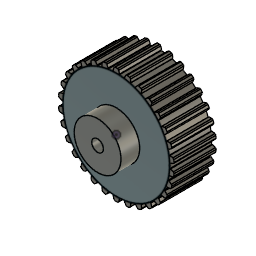
Assembly (Autodesk Fusion 360 archive; units mm, degrees)
design "Gear(30)"
part number: 2026-07-17-20-20-12-851
Autodesk Fusion 360 part; units mm, degrees
sketch "Sketch1" plane through (0, 0, 0) normal (0, 1, 0) x (1, 0, 0)
  circle A0 centre (0, 0) radius 22.8
  dimension "d1" = 45.6
  constraint coincident A0.centre origin
  measures "d1" diameter of A0
extrude "Extrude1" add sketch "Sketch1" along normal blind 18 makes body 1
sketch "Sketch2" plane through (0, 0, 0) normal (0, -1, 0) x (1, 0, 0)
  circle A0 centre (0, 0) radius 22.8
  circle A1 centre (0, 0) radius 2.5
  dimension "d4" = 5
  constraint concentric A0 A1
  measures "d4" diameter of A1
extrude "Extrude2" cut sketch "Sketch2" against normal blind 65 contours A1 bodies 1
sketch "Sketch3" plane through (0, 0, 0) normal (0, -1, 0) x (1, 0, 0)
  circle A0 centre (0, 0) radius 2.5
  circle A1 centre (0, 0) radius 22.8
  circle A2 centre (0, 0) radius 10
  dimension "d7" = 20
  constraint coincident A0.centre A1.centre
  measures "d7" diameter of A2
extrude "Extrude3" add sketch "Sketch3" along normal blind 8 contours A2 bodies 1
sketch "Sketch5" plane through (0, 18, 0) normal (0, 1, 0) x (-1, 0, 0)
  circle A0 centre (0, 0) radius 2.5
  circle A1 centre (0, 0) radius 22.8
  circle A2 centre (0, 0) radius 22.8
  line L0 (-1.3883, 23.1344) -> (-1.0229, 24.3903)
  line L1 (-1.1003, 22.7506) -> (1.0933, 22.7506)
  line L2 (-0.5435, 24.7506) -> (0.5131, 24.7506)
  line L3 (0.9908, 24.3982) -> (1.3799, 23.1392)
  arc A3 (-0.5435, 24.7506) -> (-1.0229, 24.3903) centre (-0.5428, 24.2506) ccw
  arc A4 (0.9908, 24.3982) -> (0.5131, 24.7506) centre (0.5131, 24.2506) ccw
  arc A5 (-1.3883, 23.1344) -> (-1.1003, 22.7506) centre (-1.1003, 23.0506) ccw
  arc A6 (1.0933, 22.7506) -> (1.3799, 23.1392) centre (1.0933, 23.0506) ccw
  point P0 (-1.5, 22.7506)
  point P1 (-0.918, 24.7506)
  point P2 (1.5, 22.7506)
  point P3 (0.882, 24.7506)
  dimension "d28" = 3
  dimension "d29" = 1.8
  dimension "d31" = 2
  dimension "d32" = 0.5
  dimension "d33" = 0.5
  dimension "d34" = 0.3
  constraint coincident A2 P0
  constraint horizontal L1
  constraint horizontal L2
  constraint coincident A2 P2
  constraint coincident P1 L0
  constraint coincident P1 L2
  constraint tangent L0 A3
  constraint coincident P3 L2
  constraint coincident P3 L3
  constraint tangent L2 A4
  constraint tangent L3 A4
  constraint coincident P0 L0
  constraint coincident P0 L1
  constraint tangent L0 A5
  constraint tangent L1 A5
  constraint coincident P2 L1
  constraint coincident P2 L3
  constraint tangent L1 A6
  constraint tangent L3 A6
  constraint equal A5 A6
  measures "d28" distance of P0 P2
  measures "d29" distance of P1 P3
  measures "d31" distance of L1 L2
  measures "d32" radius of A3
  measures "d33" radius of A4
  measures "d34" radius of A5
extrude "Extrude7" add sketch "Sketch5" against normal blind 18 separate body contours A1 A2 L0 L2 L3 A3 A4 A5 A6 makes body 2
pattern_circular "C-Pattern3" count 30 over 360 about axis through (0, 18, 0) along (0, -1, 0) of "Extrude7" makes body 3 at (-3.8213, 6, 22.4775) makes body 4 at (-9.3924, 6, 20.7755) makes body 5 at (-13.5066, 6, 18.3688) makes body 6 at (-16.3034, 6, 15.9386) makes body 7 at (-19.8102, 6, 11.287) makes body 8 at (-21.6416, 6, 7.1751) makes body 9 at (-22.6883, 6, 2.2537) makes body 10 at (-22.6611, 6, -2.5127) makes body 11 at (-21.6435, 6, -7.1693) makes body 12 at (-20.1965, 6, -10.5802) makes body 13 at (-16.8563, 6, -15.3527) makes body 14 at (-14.1471, 6, -17.8801) makes body 15 at (-9.1545, 6, -20.8815) makes body 16 at (-5.6515, 6, -22.0885) makes body 17 at (0.1302, 6, -22.7996) makes body 18 at (4.8677, 6, -22.2743) makes body 19 at (9.3924, 6, -20.7755) makes body 20 at (12.6333, 6, -18.98) makes body 21 at (16.3034, 6, -15.9386) makes body 22 at (19.8102, 6, -11.287) makes body 23 at (21.6416, 6, -7.1751) makes body 24 at (22.6883, 6, -2.2537) makes body 25 at (22.6611, 6, 2.5127) makes body 26 at (21.6435, 6, 7.1693) makes body 27 at (20.1965, 6, 10.5802) makes body 28 at (16.8563, 6, 15.3527) makes body 29 at (14.1471, 6, 17.8801) makes body 30 at (10.1205, 6, 20.4308) makes body 31 at (5.6515, 6, 22.0885)

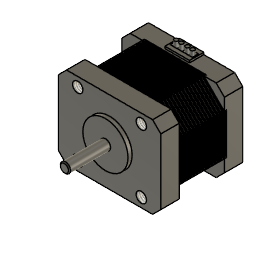
design "conveyor_belt_Assembly"
part number: 2026-07-17-14-44-36-904
Autodesk Fusion 360 part; units mm, degrees
sketch "Sketch1" plane through (0, 0, 0) normal (0, 0, 1) x (1, 0, 0)
  line L0 (25, -20) -> (-25, -20)
  line L1 (-25, -20) -> (-25, 20)
  line L2 (-25, 20) -> (25, 20)
  line L3 (25, 20) -> (25, -20)
  line L4 (25, -20) -> (-25, 20) construction
  line L5 (-25, -20) -> (25, 20) construction
  dimension "d1" = 50
  dimension "d2" = 40
  constraint horizontal L0
  constraint perpendicular L0 L1
  constraint parallel L0 L2
  constraint parallel L1 L3
  constraint coincident L4 origin
  constraint coincident L5 origin
  measures "d1" distance of L1.end L2.end
  measures "d2" distance of L0.end L1.end
extrude "Extrude1" add sketch "Sketch1" along normal blind 40
chamfer "Chamfer1" distance 4 angle 45 4 edges at (25, 0, 40) (25, 0, 0) (-25, 0, 40) (-25, 0, 0)
sketch "Sketch2" plane through (0, -20, 0) normal (0, -1, 0) x (1, 0, 0)
  line L0 (-25, 4) -> (-21, 0)
  line L1 (-21, 0) -> (21, 0)
  line L2 (21, 0) -> (25, 4)
  line L3 (25, 4) -> (25, 36)
  line L4 (25, 36) -> (21, 40)
  line L5 (21, 40) -> (-21, 40)
  line L6 (-21, 40) -> (-25, 36)
  line L7 (-25, 36) -> (-25, 4)
  circle A0 centre (0, 20) radius 2.5
  dimension "d6" = 40
  dimension "d7" = 5
  dimension "d8" = 20
  measures "d6" distance of L1 L5
  measures "d7" diameter of A0
  measures "d8" distance of origin A0.centre
extrude "Extrude2" add sketch "Sketch2" along normal blind 22 contours A0
sketch "Sketch3" plane through (0, -20, 0) normal (0, -1, 0) x (1, 0, 0)
  circle A0 centre (0, 20) radius 2.5
  line L0 (-25, 4) -> (-21, 0)
  line L1 (-21, 0) -> (21, 0)
  line L2 (21, 0) -> (25, 4)
  line L3 (25, 4) -> (25, 36)
  line L4 (25, 36) -> (21, 40)
  line L5 (21, 40) -> (-21, 40)
  line L6 (-21, 40) -> (-25, 36)
  line L7 (-25, 36) -> (-25, 4)
  circle A1 centre (0, 20) radius 11
  dimension "d12" = 22
  constraint concentric A0 A1
  measures "d12" diameter of A1
extrude "Extrude3" add sketch "Sketch3" along normal blind 2 contours A1
sketch "Sketch4" plane through (0, -20, 0) normal (0, -1, 0) x (1, 0, 0)
  circle A0 centre (0, 20) radius 11
  line L0 (-25, 4) -> (-21, 0)
  line L1 (-21, 0) -> (21, 0)
  line L2 (21, 0) -> (25, 4)
  line L3 (25, 4) -> (25, 36)
  line L4 (25, 36) -> (21, 40)
  line L5 (21, 40) -> (-21, 40)
  line L6 (-21, 40) -> (-25, 36)
  line L7 (-25, 36) -> (-25, 4)
  circle A1 centre (-15.5, 35.5) radius 2
  circle A2 centre (-15.5, 4.5) radius 2
  circle A3 centre (15.5, 4.5) radius 2
  circle A4 centre (15.5, 35.5) radius 2
  dimension "d15" = 4
  dimension "d16" = 15.5
  dimension "d17" = 15.5
  dimension "d19" = 360
  measures "d15" diameter of A1
  measures "d16" vertical distance of A0.centre A1.centre
  measures "d17" horizontal distance of A0.centre A1.centre
sketch "Sketch5" plane through (0, 20, 0) normal (0, 1, 0) x (-1, 0, 0)
  line L0 (21, 0) -> (25, 4)
  line L1 (25, 4) -> (25, 36)
  line L2 (25, 36) -> (21, 40)
  line L3 (21, 40) -> (-21, 40)
  line L4 (-21, 40) -> (-25, 36)
  line L5 (-25, 36) -> (-25, 4)
  line L6 (-25, 4) -> (-21, 0)
  line L7 (-21, 0) -> (21, 0)
  line L8 (-25, 30) -> (-15, 40)
  line L9 (-25, 30) -> (-25, 40)
  line L10 (-25, 40) -> (-15, 40)
  line L11 (25, 10) -> (15, 0)
  line L12 (25, 0) -> (15, 0)
  line L13 (25, 10) -> (25, 0)
  line L14 (-25, 10) -> (-15, 0)
  line L15 (-25, 10) -> (-25, 0)
  line L16 (-25, 0) -> (-15, 0)
  line L17 (25, 40) -> (15, 40)
  line L18 (25, 30) -> (25, 40)
  line L19 (25, 30) -> (15, 40)
  point P0 (0, 20)
  dimension "d20" = 10
  dimension "d21" = 10
  dimension "d22" = 20
  dimension "d25" = 10
  dimension "d26" = 10
  constraint coincident L5 L8.start
  constraint coincident L3 L8.end
  constraint parallel L5 L9
  constraint coincident L5 L14.start
  constraint coincident L7 L14.end
  constraint parallel L5 L15
  constraint perpendicular L15 L16
  measures "d20" distance of L3 L8.start
  measures "d21" distance of L5 L8.end
  measures "d22" distance of origin P0
  measures "d25" distance of L7 L14.start
  measures "d26" distance of L5 L14.end
extrude "Extrude4" cut sketch "Sketch5" against normal blind 22 from surface at -9 contours L0 L1 L7 L11 L12 L13 | L0 L12 L13 | L5 L6 L7 L14 L15 L16 | L1 L2 L3 L17 L18 L19 | L6 L15 L16 | L2 L17 L18 | L3 L4 L5 L8 L9 L10 | L4 L9 L10
sketch "Sketch6" plane through (0, 11, 0) normal (0, -1, 0) x (1, 0, 0)
  line L0 (25, 36) -> (21, 40)
  line L1 (21, 40) -> (15, 40)
  line L2 (15, 40) -> (25, 30)
  line L3 (25, 30) -> (25, 36)
  line L4 (-25, 10) -> (-15, 0)
  line L5 (-15, 40) -> (15, 40)
  line L6 (-25, 10) -> (-25, 30)
  line L7 (25, 10) -> (15, 0)
  line L8 (25, 30) -> (15, 40)
  line L9 (-15, 0) -> (15, 0)
  line L10 (15, 0) -> (25, 10)
  line L11 (25, 30) -> (25, 10)
  line L12 (25, 30) -> (15, 40)
  line L13 (-15, 40) -> (-25, 30)
  line L14 (-14.7929, 39.5) -> (14.7929, 39.5)
  line L15 (24.5, 29.7929) -> (14.7929, 39.5)
  line L16 (24.5, 29.7929) -> (24.5, 10.2071)
  line L17 (14.7929, 0.5) -> (24.5, 10.2071)
  line L18 (-14.7929, 0.5) -> (14.7929, 0.5)
  line L19 (-24.5, 10.2071) -> (-14.7929, 0.5)
  line L20 (-24.5, 10.2071) -> (-24.5, 29.7929)
  line L21 (-14.7929, 39.5) -> (-24.5, 29.7929)
  dimension "d42" = -0.5
  constraint coincident L4.start L6.start
  constraint coincident L4.end L9.start
  constraint coincident L7.end L9.end
  constraint coincident L7.start L10.end
  constraint coincident L2.end L3.start
  constraint coincident L1.end L2.start
  constraint perpendicular L2 L13
extrude "Extrude7" cut sketch "Sketch6" against normal blind 1 contours L2 L4 L5 L6 L7 L8 L9 L10 L11 L12 L13
pattern_linear "R-Pattern2" count 16 spacing 1.4667 along (0, -1, 0) of "Extrude7"
sketch "Sketch7" plane through (0, 0, 40) normal (0, 0, 1) x (-1, 0, 0)
  line L0 (15, -11) -> (15, -12)
  line L1 (15, -12) -> (-15, -12)
  line L2 (-15, -12) -> (-15, -11)
  line L3 (-15, -11) -> (-21, -11)
  line L4 (-21, -11) -> (-21, -20)
  line L5 (-21, -20) -> (21, -20)
  line L6 (21, -20) -> (21, -11)
  line L7 (21, -11) -> (15, -11)
  line L8 (0, -20) -> (0, -13) construction
  line L9 (-6, -20) -> (6, -20)
  line L10 (6, -20) -> (6, -13)
  line L11 (6, -13) -> (-6, -13)
  line L12 (-6, -13) -> (-6, -20)
  line L13 (-6, -20) -> (6, -13) construction
  line L14 (6, -20) -> (-6, -13) construction
  point P0 (0, -16.5)
  dimension "d49" = 12
  constraint midpoint L5 L8.start
  constraint perpendicular L5 L8
  constraint horizontal L9
  constraint perpendicular L9 L10
  constraint parallel L9 L11
  constraint parallel L10 L12
  constraint coincident L13 P0
  constraint coincident L14 P0
  constraint midpoint L8 P0
  measures "d49" distance of L10.end L11.end
extrude "Extrude8" add sketch "Sketch7" along normal blind 1 contours L5 L9 L10 L11 L12
sketch "Sketch8" plane through (0, 0, 41) normal (0, 0, 1) x (-1, 0, 0)
  line L0 (-6, -13) -> (-6, -20)
  line L1 (-6, -20) -> (6, -20)
  line L2 (6, -20) -> (6, -13)
  line L3 (6, -13) -> (-6, -13)
  line L4 (0, -20) -> (0, -13) construction
  circle A0 centre (4, -16.5224) radius 1
  circle A1 centre (1.5, -16.5224) radius 1
  circle A2 centre (-1.5, -16.5015) radius 1
  circle A3 centre (-4, -16.5015) radius 1
  line L5 (5.43, -18.0262) -> (5.43, -15)
  line L6 (5.43, -15) -> (-5.43, -15)
  line L7 (-5.43, -15) -> (-5.43, -17.9978)
  line L8 (-5.43, -17.9978) -> (5.43, -18.0262)
  dimension "d52" = 2
  dimension "d53" = 2
  dimension "d54" = 2
  dimension "d55" = 2
  dimension "d56" = 1.5
  dimension "d57" = 1.5
  dimension "d58" = 2.5
  dimension "d59" = 2
  dimension "d60" = 2.5
  dimension "d61" = 0.57
  dimension "d62" = 0.57
  dimension "d63" = 0.15
  dimension "d64" = 2
  dimension "d65" = 1.5
  dimension "d66" = 1.5
  constraint midpoint L1 L4.start
  constraint midpoint L3 L4.end
  constraint parallel L2 L5
  constraint perpendicular L4 L6
  constraint perpendicular L6 L7
  measures "d52" diameter of A0
  measures "d53" diameter of A1
  measures "d54" diameter of A2
  measures "d55" diameter of A3
  measures "d56" distance of L4 A1.centre
  measures "d57" distance of L4 A2.centre
  measures "d58" distance of A2.centre A3.centre
  measures "d59" distance of L0 A3.centre
  measures "d60" distance of A0.centre A1.centre
  measures "d61" distance of L2 L5
  measures "d62" distance of L0 L7
  measures "d63" angle of L1 L8
  measures "d64" distance of L4.end L6
  measures "d65" distance of A0.centre L8
  measures "d66" distance of A3.centre L8
extrude "Extrude9" cut sketch "Sketch8" against normal blind 1 contours L5 L6 L7 L8
extrude "Extrude10" add 4 faces at (-3.8533, 16.169, 41) (-1.5742, 16.818, 41) (1.5742, 16.2059, 41) (3.7374, 16.5176, 41) along direction (0, 0, 1) blind 2
chamfer "Chamfer2" distance 0.5 angle 45 1 edges at (-2.3308, -42, 19.096)
hole "Hole1" at (15.5, -20, 35.5) at (-15.5, -20, 35.5) at (-15.5, -20, 4.5) at (15.5, -20, 4.5) direction (0, 1, 0) diameter 5.035 depth 5 tip angle 118
thread "Thread1" "ISO Metric profile 6.0 M6x1 M6x1 6H" thread offset 0 thread depth 7.4
ref_plane "WorkPlane1" through (0, -32, 20) normal (0, -1, 0) x (1, 0, 0)
